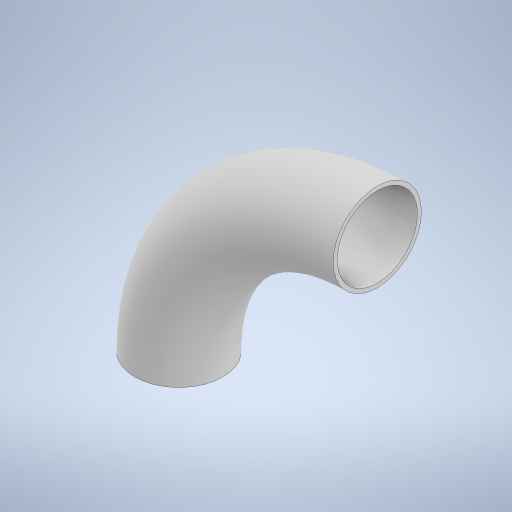
# Autodesk Inventor part: 06-01-2023 curva 90° R200
Saved by Autodesk Inventor 2023 (Build 270158000, 158)
## iProperties
Created: 2023-06-01
Part Number: 06-01-2023 curva 90° R200
Material: Generico
Document SubType Name: Modeling
Designer: Admin
Density: 1 g/cm^3
Appearance: Default
Author: Admin
Autodesk Inventor part; units mm, degrees
ref_plane "YZ Plane" through (0, 0, 0) normal (1, 0, 0) x (0, 1, 0)
ref_plane "XZ Plane" through (0, 0, 0) normal (0, 1, 0) x (-1, 0, 0)
ref_plane "XY Plane" through (0, 0, 0) normal (0, 0, 1) x (1, 0, 0)
sketch "Schizzo1" plane through (0, 0, 0) normal (0, 1, 0) x (-1, 0, 0)
  circle A0 centre (0, 0) radius 44.45
  circle A1 centre (0, 0) radius 40.45
  dimension "d0" = 88.9
  dimension "d1" = 4
  constraints: 2 centre point, 2 coincident
  measures "d0" diameter of A0
  measures "d1" radial gap between concentric circles of A0 A1
sketch "Schizzo2" plane through (0, 0, 0) normal (0, 0, 1) x (1, 0, 0)
  arc A0 (200, 200) -> (0, 0) centre (200, 0) ccw
  line L0 (200, 0) -> (200, 200) construction
  line L1 (200, 0) -> (0, 0) construction
  dimension "d3" = 200
  dimension "d4" = 90
  constraints: 4 end point, 2 point on circle, 1 centre point, 1 horizontal alignment
  measures "d3" distance of L0.start L0.end
sweep "Sweep1" add profiles "Schizzo1" path "Schizzo2"
